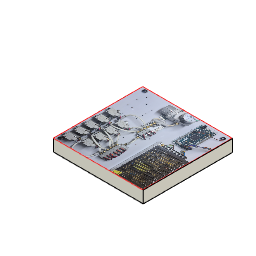
SoftControl_assembly v2 (Autodesk Fusion 360 archive; units mm, degrees)
design "Robot_version_final_assembly_Banco_neumatico"
Autodesk Fusion 360 part; units mm, degrees
sketch "Boceto1" plane through (0, 510, 0) normal (0, 1, 0) x (-1, 0, 0)
  line L0 (250, -244.5) -> (-250, -244.5)
  line L1 (-250, -244.5) -> (-250, -252)
  line L2 (-250, -252) -> (250, -252)
  line L3 (250, -252) -> (250, -244.5)
  line L4 (0, 0) -> (0, -321.9026)
  line L5 (150, -246.5086) -> (-150, -246.5086)
  line L6 (-150, -246.5086) -> (-150, 53.4914)
  line L7 (-150, 53.4914) -> (150, 53.4914)
  line L8 (150, 53.4914) -> (150, -246.5086)
  line L9 (150, -246.5086) -> (-150, 53.4914) construction
  line L10 (-150, -246.5086) -> (150, 53.4914) construction
  point P0 (0, -96.5086)
  dimension "d723" = 300
  dimension "d724" = 300
  constraint coincident L4.start origin
  constraint perpendicular L0 L4
  constraint horizontal L5
  constraint perpendicular L5 L6
  constraint parallel L5 L7
  constraint parallel L6 L8
  constraint coincident L9 P0
  constraint coincident L10 P0
  constraint coincident L4 P0
  measures "d723" distance of L6.end L7.end
  measures "d724" distance of L5.end L6.end
extrude "Extruir1" add sketch "Boceto1" along normal blind 40 contours L0 L6 L7 L8

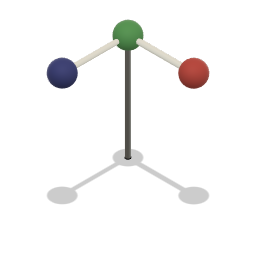
design "bolas_luminosas"
Autodesk Fusion 360 part; units mm, degrees
sketch "Boceto1" plane through (0, -14.7, 0) normal (0, -1, 0) x (1, 0, 0)
  arc A0 (11.1086, 24.3893) -> (-11.1086, 24.3893) centre (0, 0) ccw
  arc A1 (-5.3435, 19.9423) -> (-11.1086, 24.3893) centre (-11.1391, 18.3894) ccw
  line L0 (-5.3435, 19.9423) -> (-2.0867, 7.7875)
  arc A2 (-3.3058, 3.7513) -> (-2.0867, 7.7875) centre (-5.9504, 6.7523) ccw
  arc A3 (-3.3058, 3.7513) -> (-4.9016, 0.9872) centre (0, 0) ccw
  arc A4 (-7.7875, -2.0867) -> (-4.9016, 0.9872) centre (-8.8228, 1.777) ccw
  line L1 (-7.7875, -2.0867) -> (-19.9423, -5.3435)
  arc A5 (-26.6761, -2.5744) -> (-19.9423, -5.3435) centre (-21.4952, 0.452) ccw
  arc A6 (-26.6761, -2.5744) -> (-16.0884, -21.4337) centre (0, 0) ccw
  arc A7 (-14.8196, -14.8196) -> (-16.0884, -21.4337) centre (-10.5769, -19.0622) ccw
  line L2 (-14.8196, -14.8196) -> (-5.7009, -5.7009)
  arc A8 (-1.5958, -4.7385) -> (-5.7009, -5.7009) centre (-2.8725, -8.5293) ccw
  arc A9 (-1.5958, -4.7385) -> (1.5958, -4.7385) centre (0, 0) ccw
  arc A10 (5.7009, -5.7009) -> (1.5958, -4.7385) centre (2.8725, -8.5293) ccw
  line L3 (5.7009, -5.7009) -> (14.8196, -14.8196)
  arc A11 (16.0884, -21.4337) -> (14.8196, -14.8196) centre (10.5769, -19.0622) ccw
  arc A12 (16.0884, -21.4337) -> (26.6761, -2.5744) centre (0, 0) ccw
  arc A13 (19.9423, -5.3435) -> (26.6761, -2.5744) centre (21.4952, 0.452) ccw
  line L4 (19.9423, -5.3435) -> (7.7875, -2.0867)
  arc A14 (4.9016, 0.9872) -> (7.7875, -2.0867) centre (8.8228, 1.777) ccw
  arc A15 (4.9016, 0.9872) -> (3.3058, 3.7513) centre (0, 0) ccw
  arc A16 (2.0867, 7.7875) -> (3.3058, 3.7513) centre (5.9504, 6.7523) ccw
  line L5 (2.0867, 7.7875) -> (5.3435, 19.9423)
  arc A17 (11.1086, 24.3893) -> (5.3435, 19.9423) centre (11.1391, 18.3894) ccw
  circle A18 centre (0, 0) radius 1.75
  circle A19 centre (0, 0) radius 1.5
  circle A20 centre (0, 0) radius 1.75
  dimension "d727" = 3
  constraint concentric A0 A19
  constraint concentric A0 A20
  measures "d727" diameter of A19
extrude "Extruir1" add sketch "Boceto1" along normal blind 68.963 contours A19 makes body 1
sketch "Boceto2" plane through (0, 0, 0) normal (0, 0, 1) x (1, 0, 0)
  circle A0 centre (0.0192, 36.2772) radius 1.4742
  circle A1 centre (0.0192, 36.2772) radius 7.5
  line L0 (0.0192, 36.2772) -> (0.0192, 43.7772)
  line L1 (0.0192, 36.2772) -> (45.0192, 36.2772)
  circle A2 centre (45.0192, 36.2772) radius 7.5
  line L2 (45.0192, 36.2772) -> (45.0192, 43.7772)
  line L3 (0.0192, 36.2772) -> (0.0192, 43.7772)
  line L4 (0.0192, 43.7772) -> (0.0192, 28.7772)
  line L5 (45.0192, 43.7772) -> (45.0192, 28.7772)
  dimension "d730" = 15
  dimension "d731" = 45
  dimension "d732" = 15
  constraint concentric A0 A1
  constraint coincident A0.centre A1.centre
  constraint coincident A1 L0.end
  constraint vertical L0
  constraint perpendicular L0 L1
  constraint coincident L1.end A2.centre
  constraint coincident A2 L2.end
  constraint perpendicular L1 L2
  constraint coincident A1 L4.end
  constraint parallel L0 L4
  constraint coincident A2 L5.end
  constraint perpendicular L1 L5
  measures "d730" diameter of A1
  measures "d731" distance of A0.centre L1.end
  measures "d732" diameter of A2
extrude "Extruir2" add sketch "Boceto2" along normal blind 45 contours A0 L0 L1 L3 L4 | A0 L1 L4 | A0 L0 L3 L4 bodies 1 makes body 2
sketch "Boceto3" plane through (0, 0, 0) normal (1, 0, 0) x (0, 0, -1)
  circle A0 centre (-0.1215, 36.3898) radius 1.6927
extrude "Extruir3" add sketch "Boceto3" along normal blind 45 bodies 2 1
sketch "Boceto4" plane through (0, 0, 0) normal (1, 0, 0) x (0, 0, -1)
  circle A0 centre (-44.9136, 36.2943) radius 7.5
  line L0 (-44.9136, 36.2943) -> (-44.9136, 43.7943)
  line L1 (-44.9136, 43.7943) -> (-44.9136, 28.7943)
  dimension "d737" = 15
  constraint coincident A0.centre L0.start
  constraint coincident A0 L0.end
  constraint vertical L0
  constraint coincident A0 L1.end
  constraint parallel L0 L1
  measures "d737" diameter of A0
revolve "Revolución1" add sketch "Boceto4" angle 360 about axis through (0, 43.7943, 44.9136) along (0, -1, 0) separate body contours A0 L0 L1 picked at (-48.0224, 32.3961) makes body 3
revolve "Revolución2" add sketch "Boceto2" angle 360 about axis through (0.0192, 43.7772, 0) along (0, -1, 0) separate body contours A0 A1 L0 L3 L4 makes body 4
revolve "Revolución3" add sketch "Boceto2" angle 360 about axis through (45.0192, 36.2772, 0) along (0, 1, 0) separate body contours A2 L2 L5 makes body 5
move_body "Verschieben1" bodies 5 4 3 2 to x (1, 0, 0) y (0, 1, 0) z (0, 0, 1) at (0, -47.5341, 0)
